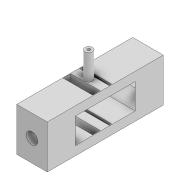
# Autodesk Inventor part: 20220727_1cell_PBME
Saved by Autodesk Inventor 2022 (Build 260153000, 153)
## iProperties
Created: 2022-07-28
Part Number: 20220727_1cell_PBME
Material: Generic
Document SubType Name: Modeling
Designer: scott
Density: 1 g/cm^3
Appearance: Default
Author: scott
Autodesk Inventor part; units mm, degrees
ref_plane "YZ Plane" through (0, 0, 0) normal (1, 0, 0) x (0, 1, 0)
ref_plane "XZ Plane" through (0, 0, 0) normal (0, 1, 0) x (-1, 0, 0)
ref_plane "XY Plane" through (0, 0, 0) normal (0, 0, 1) x (1, 0, 0)
sketch "Sketch1" plane through (0, 0, 0) normal (0, 1, 0) x (-1, 0, 0)
  line L0 (0, 0) -> (-24, 0)
  line L1 (-24, 0) -> (-24, -91)
  line L2 (-24, -91) -> (0, -91)
  line L3 (0, -91) -> (0, 0)
  dimension "d0" = 91
  dimension "d1" = 24
  constraints: 8 end point, 2 parallel, 1 horizontal, 1 perpendicular
  measures "d0" distance of L0.end L1.end
  measures "d1" distance of L1.end L2.end
extrude "Extrusion1" add sketch "Sketch1" along normal blind 34
sketch "Sketch2" plane through (24, 0, 0) normal (1, 0, 0) x (0, 0, -1)
  line L0 (22, 27) -> (69, 27)
  line L1 (69, 27) -> (69, 7)
  line L2 (69, 7) -> (22, 7)
  line L3 (22, 7) -> (22, 27)
  line L4 (0, 34) -> (91, 34) projected
  line L5 (0, 0) -> (91, 0) projected
  line L6 (0, 0) -> (0, 34) projected
  line L7 (91, 0) -> (91, 34) projected
  dimension "d4" = 7
  dimension "d5" = 7
  dimension "d6" = 22
  dimension "d7" = 22
  constraints: 8 end point, 2 parallel, 1 horizontal, 1 perpendicular
  measures "d4" distance between parallel lines of L4 L0
  measures "d5" distance between parallel lines of L5 L2
  measures "d6" distance between parallel lines of L6 L3
  measures "d7" distance between parallel lines of L7 L1
extrude "Extrusion2" cut sketch "Sketch2" against normal up to surface (24 mm away) contours L0 L1 L2 L3
sketch "Sketch3" plane through (0, 34, 0) normal (0, 1, 0) x (1, 0, 0)
  line L0 (0.5, 42) -> (23.5, 42)
  line L1 (23.5, 42) -> (23.5, 36)
  line L2 (23.5, 36) -> (0.5, 36)
  line L3 (0.5, 36) -> (0.5, 42)
  line L4 (0, 91) -> (0, 0) projected
  line L5 (24, 0) -> (24, 91) projected
  line L6 (0, 0) -> (24, 0) projected
  dimension "d10" = 0.5
  dimension "d11" = 0.5
  dimension "d12" = 6
  dimension "d13" = 36
  constraints: 8 end point, 2 parallel, 1 horizontal, 1 perpendicular
  measures "d10" distance between parallel lines of L4 L3
  measures "d11" distance between parallel lines of L5 L1
  measures "d12" distance between parallel lines of L2 L0
  measures "d13" distance between parallel lines of L6 L2
extrude "Extrusion3" cut sketch "Sketch3" against normal up to surface (34 mm away)
sketch "Sketch4" plane through (0, 34, 0) normal (0, 1, 0) x (1, 0, 0)
  line L0 (0.5, 51) -> (23.5, 51)
  line L1 (23.5, 51) -> (23.5, 49)
  line L2 (23.5, 49) -> (0.5, 49)
  line L3 (0.5, 49) -> (0.5, 51)
  line L4 (0.5, 42) -> (23.5, 42) projected
  line L5 (24, 0) -> (24, 91) projected
  line L6 (0, 91) -> (0, 0) projected
  dimension "d16" = 2
  dimension "d17" = 7
  dimension "d18" = 0.5
  dimension "d19" = 0.5
  constraints: 8 end point, 2 parallel, 1 horizontal, 1 perpendicular
  measures "d16" distance of L0.end L1.end
  measures "d17" distance between parallel lines of L4 L2
  measures "d18" distance between parallel lines of L5 L1
  measures "d19" distance between parallel lines of L6 L3
extrude "Extrusion4" cut sketch "Sketch4" against normal up to surface (34 mm away)
sketch "Sketch5" plane through (0, 0, 0) normal (0, 0, 1) x (1, 0, 0)
  circle A0 centre (12, 17) radius 4.5
  line L0 (0, 0) -> (24, 0) projected
  line L1 (24, 0) -> (24, 34) projected
  dimension "d22" = 17
  dimension "d23" = 12
  dimension "d24" = 9
  constraints: 1 centre point
  measures "d22" distance from line of L0 A0.centre
  measures "d23" distance from line of L1 A0.centre
  measures "d24" diameter of A0
extrude "Extrusion5" cut sketch "Sketch5" against normal blind 12
loft "Loft1" cut section 1 edges at (7.5, 17, -12) section 2 edges at (0, 17, -22) (12, 27, -22) (24, 17, -22) (12, 7, -22)
sketch "Sketch6" plane through (24, 0, -91) normal (0, 0, -1) x (-1, 0, 0)
  circle A0 centre (12, 17) radius 4.5
  line L0 (24, 0) -> (24, 34) projected
  line L1 (0, 0) -> (24, 0) projected
  dimension "d31" = 12
  dimension "d32" = 17
  dimension "d33" = 9
  constraints: 1 centre point
  measures "d31" distance from line of L0 A0.centre
  measures "d32" distance from line of L1 A0.centre
  measures "d33" diameter of A0
extrude "Extrusion6" cut sketch "Sketch6" against normal blind 12
loft "Loft2" cut section 1 edges at (16.5, 17, -79) section 2 edges at (0, 17, -69) (12, 7, -69) (24, 17, -69) (12, 27, -69)
sketch "Sketch7" plane through (0, 34, 0) normal (0, 1, 0) x (1, 0, 0)
  circle A0 centre (11, 45.5) radius 3
  line L0 (0, 91) -> (0, 0) projected
  line L1 (24, 0) -> (24, 91) projected
  line L2 (0.5, 42) -> (23.5, 42) projected
  line L3 (23.5, 49) -> (0.5, 49) projected
  dimension "d40" = 11
  dimension "d41" = 13
  dimension "d42" = 3.5
  dimension "d43" = 3.5
  dimension "d44" = 6
  constraints: 1 centre point
  measures "d40" distance from line of L0 A0.centre
  measures "d41" distance from line of L1 A0.centre
  measures "d42" distance from line of L2 A0.centre
  measures "d43" distance from line of L3 A0.centre
  measures "d44" diameter of A0
extrude "Extrusion7" add sketch "Sketch7" along normal blind 20
sketch "Sketch8" plane through (11, 54, -45.5) normal (0, 1, 0) x (1, 0, 0)
  circle A0 centre (0, 0) radius 1.25
  point P0 (-11, -45.5)
  dimension "d47" = 2.5
  constraints: 1 centre point
  measures "d47" diameter of A0
extrude "Extrusion8" cut sketch "Sketch8" against normal up to surface (27 mm away)
body "Solid1"
